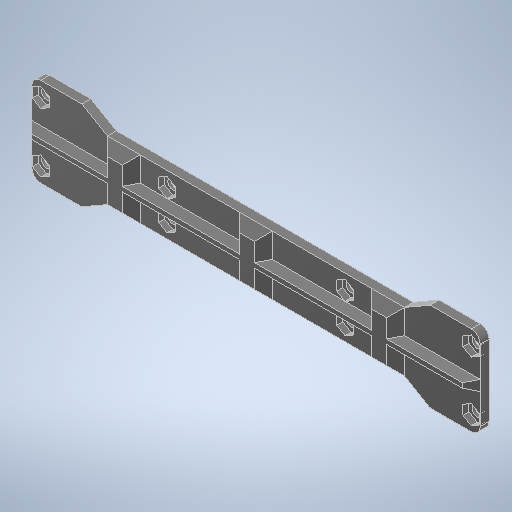
# Autodesk Inventor part: 3D_frame-connect-base3
Saved by Autodesk Inventor 2025 (Build 290162000, 162)
## iProperties
Created: 2024-07-30
Part Number: 3D_frame-connect-base3
Material: 一般
Document SubType Name: Modeling
Designer: 8326d
Density: 1 g/cm^3
Appearance: 滑らか - 黒
Author: 8326d
## iProperties of the stored document 3D_frame-connect-base3_3D プリント.ipt
Created: 2024-08-06
Part Number: 3D_frame-connect-base3_3D プリント
Material: 一般
Document SubType Name: Modeling
Designer: 8326d
Density: 1 g/cm^3
Appearance: 既定
Author: 8326d
Autodesk Inventor part; units mm, degrees
ref_plane "YZ Plane" through (0, 0, 0) normal (1, 0, 0) x (0, 1, 0)
ref_plane "XZ Plane" through (0, 0, 0) normal (0, 1, 0) x (-1, 0, 0)
ref_plane "XY Plane" through (0, 0, 0) normal (0, 0, 1) x (1, 0, 0)
sketch "スケッチ1" plane through (0, 0, 0) normal (0, 0, 1) x (1, 0, 0)
  line L0 (-75.5, -15) -> (75.5, -15)
  line L1 (75.5, -15) -> (75.5, 15)
  line L2 (75.5, 15) -> (-75.5, 15)
  line L3 (-75.5, 15) -> (-75.5, -15)
  line L4 (-75.5, -15) -> (75.5, 15) construction
  line L5 (75.5, -15) -> (-75.5, 15) construction
  point P0 (0, 0)
  dimension "d0" = 151
  dimension "d1" = 30
  constraints: 12 end point, 2 midpoint, 2 parallel, 1 horizontal, 1 perpendicular
  measures "d0" distance of L2.end L1.end
  measures "d1" distance of L1.end L0.end
extrude "押し出し1" add sketch "スケッチ1" along normal blind 3
sketch "スケッチ2" plane through (0, 0, 3) normal (0, 0, 1) x (1, 0, 0)
  line L0 (75.5, 15) -> (-75.5, 15) projected
  line L1 (-58.6603, 15) -> (-50, 10)
  line L2 (-50, 10) -> (50, 10)
  line L3 (50, 10) -> (58.6603, 15)
  point P0 (0, 0)
  point P1 (0, 10)
  dimension "d4" = 10
  dimension "d5" = 100
  dimension "d6" = 30
  dimension "d7" = 30
  constraints: 6 end point, 2 point on line, 1 horizontal, 1 midpoint, 1 vertical alignment
  measures "d4" distance from line of point (0, 0) L2
  measures "d5" distance of L1.end L2.end
  measures "d6" angle of L0 L1
  measures "d7" angle of L0 L3
extrude "押し出し2" cut sketch "スケッチ2" against normal through all
sketch "スケッチ3" plane through (0, 0, 3) normal (0, 0, 1) x (1, 0, 0)
  line L0 (72.5, -10) -> (-72.5, -10) construction
  line L1 (-72.5, -10) -> (-72.5, 10) construction
  line L2 (-72.5, 10) -> (72.5, 10) construction
  line L3 (72.5, 10) -> (72.5, -10) construction
  line L4 (72.5, -10) -> (-72.5, 10) construction
  line L5 (-72.5, -10) -> (72.5, 10) construction
  line L6 (30, -5) -> (-30, -5) construction
  line L7 (-30, -5) -> (-30, 5) construction
  line L8 (-30, 5) -> (30, 5) construction
  line L9 (30, 5) -> (30, -5) construction
  line L10 (30, -5) -> (-30, 5) construction
  line L11 (-30, -5) -> (30, 5) construction
  point P0 (0, 0)
  dimension "d10" = 145
  dimension "d11" = 20
  dimension "d12" = 60
  dimension "d13" = 10
  constraints: 24 end point, 4 midpoint, 4 parallel, 2 horizontal, 2 perpendicular
  measures "d10" distance of L1.end L2.end
  measures "d11" distance of L0.end L1.end
  measures "d12" distance of L7.end L8.end
  measures "d13" distance of L6.end L7.end
hole "穴1" at (-72.5, 10, 3) at (-30, 5, 3) direction (0, 0, -1) diameter 3.5 end through all
sketch "スケッチ4" plane through (0, 0, 3) normal (0, 0, 1) x (1, 0, 0)
  line L0 (-72.5, 13.2332) -> (-69.7, 11.6166)
  line L1 (-69.7, 11.6166) -> (-69.7, 8.3834)
  line L2 (-69.7, 8.3834) -> (-72.5, 6.7668)
  line L3 (-72.5, 6.7668) -> (-75.3, 8.3834)
  line L4 (-75.3, 8.3834) -> (-75.3, 11.6166)
  line L5 (-75.3, 11.6166) -> (-72.5, 13.2332)
  line L6 (-30, 8.2332) -> (-27.2, 6.6166)
  line L7 (-27.2, 6.6166) -> (-27.2, 3.3834)
  line L8 (-27.2, 3.3834) -> (-30, 1.7668)
  line L9 (-30, 1.7668) -> (-32.8, 3.3834)
  line L10 (-32.8, 3.3834) -> (-32.8, 6.6166)
  line L11 (-32.8, 6.6166) -> (-30, 8.2332)
  point P0 (0, 0)
  point P1 (-72.5, 10)
  point P2 (-30, 5)
  point P3 (-72.5, 10)
  point P4 (-30, 5)
  dimension "d42" = 5.6
  dimension "d43" = 5.6
  constraints: 24 end point, 2 coincident, 2 vertical alignment, 26 other
  measures "d42" distance between parallel lines of L4 L1
  measures "d43" distance between parallel lines of L7 L10
extrude "押し出し3" cut sketch "スケッチ4" against normal blind 2
mirror "ミラー1" about plane through (0, 0, 0) normal (1, 0, 0) of "穴1", "押し出し3"
mirror "ミラー2" about plane through (0, 0, 0) normal (0, 1, 0) of "押し出し2", "穴1", "押し出し3", "ミラー1"
sketch "スケッチ5" plane through (-75.5, -15, 0) normal (-1, 0, 0) x (0, 0, 1)
  line L0 (3, 30) -> (3, 0) projected
  line L1 (3, 16.7668) -> (6, 15.8)
  line L2 (6, 15.8) -> (6, 14.2)
  line L3 (6, 14.2) -> (3, 13.2332)
  line L4 (3, 16.7668) -> (1, 16.7668) projected
  line L5 (3, 13.2332) -> (1, 13.2332) projected
  point P0 (0, 15)
  point P1 (6, 15)
  point P2 (3, 15)
  dimension "d25" = 3
  dimension "d26" = 1.6
  constraints: 6 end point, 2 midpoint, 1 horizontal alignment
  measures "d25" distance between parallel lines of L0 L2
  measures "d26" distance of L1.end L2.end
extrude "押し出し4" add sketch "スケッチ5" against normal up to surface (151 mm away)
sketch "スケッチ6" plane through (-50, -10, 0) normal (0, -1, 0) x (1, 0, 0)
  line L0 (0, 3) -> (100, 3) projected
  line L1 (44.5, 3) -> (47.5, 6)
  line L2 (-25.5, 6) -> (125.5, 6) projected
  line L3 (52.5, 6) -> (55.5, 3)
  line L4 (100, 0) -> (0, 0) projected
  point P0 (50, 0)
  point P1 (50, 0)
  point P2 (50, 0)
  dimension "d29" = 2.5
  dimension "d30" = 2.5
  dimension "d31" = 45
  dimension "d32" = 45
  constraints: 4 end point, 4 point on line, 2 midpoint
  measures "d29" horizontal distance of L1.end point (50, 0)
  measures "d30" horizontal distance of point (50, 0) L3.start
  measures "d31" angle of L0 L1
  measures "d32" angle of L0 L3
extrude "押し出し5" add sketch "スケッチ6" against normal up to surface (20 mm away)
pattern_linear "矩形状パターン1" count 3 spacing 44.5 along (1, 0, 0) of "押し出し5" first direction both ways yes
chamfer "面取り1" distance 3 angle 45 8 edges at (-44.5, -10, 6) (-44.5, 10, 6) (0, 10, 6) (0, -10, 6) (44.5, -10, 6) (44.5, 10, 6) (-75.5, 0, 6) (75.5, 0, 6)
fillet "フィレット1" radius 3 4 edges at (-75.5, -15, 1.5) (-75.5, 15, 1.5) (75.5, -15, 1.5) (75.5, 15, 1.5)
equation "\"d7\" = d6"
equation "\"d43\" = d42"
equation "\"d30\" = d29"
equation "\"d32\" = d31"
